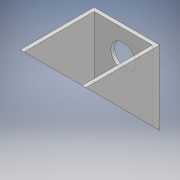
# Autodesk Inventor part: 車軸受け2
Saved by Autodesk Inventor 2018 (Build 220112000, 112)
## iProperties
Created: 2017-09-14
Part Number: 車軸受け2
Material: 一般
Document SubType Name: Modeling
Designer: mura5
Density: 1 g/cm^3
Appearance: 既定
Author: mura5
Autodesk Inventor part; units mm, degrees
ref_plane "YZ Plane" through (0, 0, 0) normal (1, 0, 0) x (0, 1, 0)
ref_plane "XZ Plane" through (0, 0, 0) normal (0, 1, 0) x (-1, 0, 0)
ref_plane "XY Plane" through (0, 0, 0) normal (0, 0, 1) x (1, 0, 0)
sketch "スケッチ1" plane through (0, 0, 0) normal (0, 0, 1) x (1, 0, 0)
  line L0 (-20, -30) -> (20, -30)
  line L1 (20, -30) -> (20, 30)
  line L2 (20, 30) -> (-20, 30)
  line L3 (-20, 30) -> (-20, -30)
  line L4 (-20, -30) -> (20, 30) construction
  line L5 (20, -30) -> (-20, 30) construction
  line L6 (-17.7, 27.7) -> (17.7, 27.7)
  line L7 (17.7, 27.7) -> (17.7, -27.7)
  line L8 (17.7, -27.7) -> (-17.7, -27.7)
  line L9 (-17.7, -27.7) -> (-17.7, 27.7)
  point P0 (0, 0)
  dimension "d0" = 40
  dimension "d1" = 60
  dimension "d2" = 2.3
  constraints: 20 end point, 4 parallel, 2 midpoint, 2 perpendicular, 1 horizontal, 3 other
  measures "d0" distance of L2.end L1.end
  measures "d1" distance of L1.end L0.end
  measures "d2" distance between parallel lines of L2 L6
extrude "押し出し1" add sketch "スケッチ1" along normal mid plane 60
chamfer "面取り1" distance 60 angle 45 1 edges at (0, -30, -30)
sketch "スケッチ2" plane through (-20, 30, 30) normal (0, 1, 0) x (1, 0, 0)
  point P0 (20, 30)
  point P1 (20, 30)
  constraints: 1 coincident
hole "穴1" at (0, 30, 0) direction (0, -1, 0) diameter 15 depth 8 tip angle 118
sketch "スケッチ4" plane through (-20, 30, 30) normal (0, 1, 0) x (1, 0, 0)
  line L0 (0, 0) -> (40, 0)
  line L1 (40, 0) -> (40, 15)
  line L2 (40, 15) -> (0, 15)
  line L3 (0, 15) -> (0, 0)
  point P0 (20, 30)
  dimension "d15" = 40
  dimension "d16" = 15
  constraints: 8 end point, 2 parallel, 1 horizontal, 1 perpendicular
  measures "d15" distance of L2.end L1.end
  measures "d16" distance of L1.end L0.end
extrude "押し出し2" cut sketch "スケッチ4" against normal blind 80
